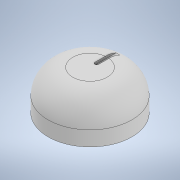
# Autodesk Inventor part: knob
Saved by Autodesk Inventor 2022 (Build 260153000, 153)
## iProperties
Created: 2021-08-07
Part Number: knob
Material: Generic
Document SubType Name: Modeling
Designer: RNG3nius
Density: 1 g/cm^3
Appearance: Default
Author: RNG3nius
Autodesk Inventor part; units mm, degrees
ref_plane "YZ Plane" through (0, 0, 0) normal (1, 0, 0) x (0, 1, 0)
ref_plane "XZ Plane" through (0, 0, 0) normal (0, 1, 0) x (-1, 0, 0)
ref_plane "XY Plane" through (0, 0, 0) normal (0, 0, 1) x (1, 0, 0)
sketch "Sketch1" plane through (0, 0, 0) normal (0, 1, 0) x (-1, 0, 0)
  circle A0 centre (0, 0) radius 17
  dimension "d0" = 34
  constraints: 1 centre point, 1 coincident
  measures "d0" diameter of A0
extrude "Extrusion1" add sketch "Sketch1" along normal blind 13
chamfer "Chamfer1" distance 4 angle 45 1 edges at (17, 13, 0)
sketch "Sketch2" plane through (0, 13, 0) normal (0, 1, 0) x (1, 0, 0)
  line L0 (0.75, 2) -> (-0.75, 2)
  line L1 (-0.75, 2) -> (-0.75, 12)
  line L2 (-0.75, 12) -> (0.75, 12)
  line L3 (0.75, 12) -> (0.75, 2)
  circle A0 centre (0, 0) radius 17 projected
  dimension "d6" = 1.5
  dimension "d7" = 10
  dimension "d8" = 2
  dimension "d9" = 16.25
  constraints: 8 end point, 2 parallel, 1 horizontal, 1 perpendicular
  measures "d6" distance of L1.end L2.end
  measures "d7" distance of L0.end L1.end
  measures "d8" distance from line of L0 point (0, 0)
  measures "d9" distance edge to line of A0 L3
extrude "Extrusion2" cut sketch "Sketch2" against normal blind 1 contours L0 L1 L2 L3
fillet "Fillet1" radius 0.75 4 edges at (0.75, 12.5, -12) (-0.75, 12.5, -12) (-0.75, 12.5, -2) (0.75, 12.5, -2)
sketch "Sketch3" plane through (0, 0, 0) normal (0, -1, 0) x (1, 0, 0)
  circle A0 centre (0, 0) radius 2.9
  line L0 (0, 0) -> (3.3833, 0) construction
  line L1 (0, 0) -> (3.3833, 0) construction
  line L2 (0, 0) -> (2.9, 0) construction
  line L3 (0, 0) -> (2.9, 0) construction
  line L4 (0, 0) -> (2.9, 0) construction
  line L5 (0, 0) -> (-0.4833, -2.8594)
  line L6 (0, 0) -> (2.9, 0) construction
  line L7 (-0.4833, -2.8594) -> (0.4833, -2.8594)
  line L8 (0, 0) -> (-0.4833, 2.8594)
  line L9 (0, 0) -> (2.9, 0) construction
  line L10 (-0.4833, 2.8594) -> (0.4833, 2.8594)
  line L11 (0.4833, 2.8594) -> (1.1703, 2.8594) construction
  line L12 (0.4833, 2.8594) -> (0, 2.1692)
  line L13 (0.4833, 2.8594) -> (1.326, 2.8594) construction
  line L14 (0, 2.1692) -> (-0.4833, 2.8594)
  line L15 (0.4833, -2.8594) -> (0, -2.1692)
  line L16 (0.4833, -2.8594) -> (1.326, -2.8594) construction
  line L17 (0, -2.1692) -> (-0.4833, -2.8594)
  dimension "d13" = 5.8
  dimension "d50" = 99.594
  dimension "d52" = 99.594
  dimension "d54" = 125
  dimension "d55" = 125
  constraints: 36 end point, 12 horizontal, 4 equal length, 4 point on circle, 1 centre point, 1 coincident
  measures "d13" diameter of A0
  measures "d50" angle of L5 L6
  measures "d52" angle of L9 L8
  measures "d54" angle of L12 L13
  measures "d55" angle of L16 L15
extrude "Extrusion7" cut sketch "Sketch3" against normal blind 10.5 contours A0 L15 L17 L5 L8 L14 L12 | L8 L5 A0
sketch "Sketch5" plane through (0, 0, 0) normal (0, -1, 0) x (1, 0, 0)
  circle A0 centre (0, 0) radius 17
  circle A1 centre (0, 0) radius 15
  constraints: 2 centre point, 2 coincident
extrude "Extrusion8" add sketch "Sketch5" along normal blind 3
chamfer "Chamfer2" distance 0.5 angle 45 2 edges at (-2.9, 0, 0) (2.9, 0, 0)
fillet "Fillet6" radius 10 2 edges at (13, 13, 0) (17, 9, 0)
body "Solid1"
